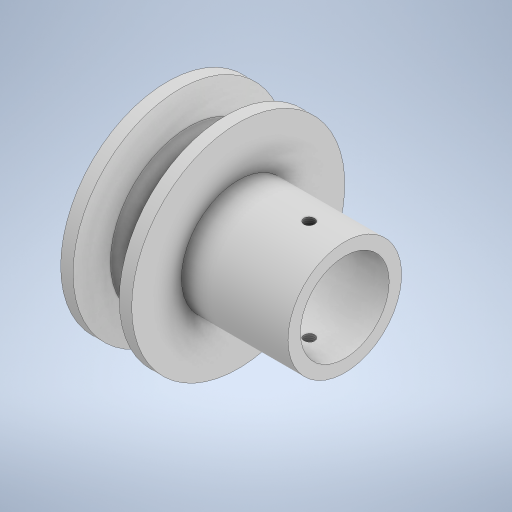
# Autodesk Inventor part: Шкив 20
Saved by Autodesk Inventor 2023 (Build 270158000, 158)
## iProperties
Created: 2022-05-01
Part Number: Шкив 20
Material: Типовые
Document SubType Name: Modeling
Designer: User
Density: 1 g/cm^3
Appearance: По умолчанию
Author: User
Autodesk Inventor part; units mm, degrees
ref_plane "YZ Plane" through (0, 0, 0) normal (1, 0, 0) x (0, 1, 0)
ref_plane "XZ Plane" through (0, 0, 0) normal (0, 1, 0) x (-1, 0, 0)
ref_plane "XY Plane" through (0, 0, 0) normal (0, 0, 1) x (1, 0, 0)
sketch "Эскиз1" plane through (0, 0, 0) normal (0, 1, 0) x (-1, 0, 0)
  line L0 (0, 30) -> (20, 30)
  line L1 (20, 30) -> (20, 0)
  line L2 (20, 0) -> (0, 0)
  line L3 (20, 30) -> (14, 30)
  line L4 (14, 30) -> (14, 22)
  line L5 (14, 22) -> (6, 22)
  line L6 (6, 22) -> (6, 30)
  line L7 (20, 0) -> (-30, 0)
  line L8 (-30, 0) -> (-30, 16)
  line L9 (-30, 16) -> (0, 16)
  line L10 (-30, 0) -> (-30, 12.5)
  line L11 (0, 16) -> (0, 30)
  line L12 (10, 22) -> (10, 30)
  line L13 (10, 30) -> (3.5, 30)
  line L14 (3.5, 30) -> (6, 22)
  line L15 (3.5, 30) -> (16.5, 30)
  line L16 (16.5, 30) -> (14, 22)
  line L17 (20, 0) -> (20, 16.5)
  line L18 (0, 0) -> (5, 0)
  line L19 (10, 16.5) -> (20, 16.5)
  line L20 (-30, 12.5) -> (10, 12.5)
  line L21 (10, 12.5) -> (10, 16.5)
  point P0 (16.5, 30)
  dimension "d0" = 30
  dimension "d1" = 20
  dimension "d2" = 6
  dimension "d3" = 8
  dimension "d4" = 8
  dimension "d5" = 50
  dimension "d6" = 16
  dimension "d7" = 12.5
  dimension "d15" = 6.5
  dimension "d16" = 13
  dimension "d23" = 16.5
  dimension "d28" = 40
  constraints: 44 end point, 10 perpendicular, 7 point on line, 2 midpoint, 1 parallel, 1 vertical
  measures "d0" distance of L2.end L0.start
  measures "d1" distance of L0.start L0.end
  measures "d2" distance of L0.end L3.end
  measures "d3" distance of L3.end L4.end
  measures "d4" distance of L4.end L5.end
  measures "d5" distance of L1.end L7.end
  measures "d6" distance of L7.end L8.end
  measures "d7" distance of L7.end L10.end
  measures "d15" distance of L12.end L13.end
  measures "d16" distance of L13.end L15.end
  measures "d23" distance of L1.end L17.end
  measures "d28" distance of L10.end L20.end
revolve "Вращение3" add sketch "Эскиз1" angle 360 about axis through (-20, 0, 0) along (1, 0, 0) contours L0 L14 L5 L16 L1 L19 L21 L20 L8 L9 L11
sketch "Эскиз3" plane through (0, 0, 0) normal (0, 1, 0) x (-1, 0, 0)
  line L0 (0, 0) -> (-30, 0)
  line L1 (-30, 16) -> (-30, -16) projected
  line L2 (-30, 0) -> (-20, 0)
  circle A0 centre (-20, 0) radius 1.5
  dimension "d30" = 10
  dimension "d31" = 3
  constraints: 4 end point, 1 centre point, 1 coincident, 1 midpoint, 1 point on line
  measures "d30" distance of L0.end L2.end
  measures "d31" diameter of A0
extrude "Выдавливание3" cut sketch "Эскиз3" along normal mid plane 153
thread "Резьба2" size "M3x0.5" class "6H" standard "ANSI Metric M Profile" full length
